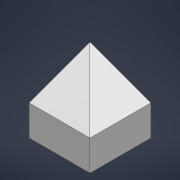
# Autodesk Inventor part: 110033226_ipt_35_中心城堡圍牆頂部_MIR
Saved by Autodesk Inventor 2022 (Build 260153000, 153)
## iProperties
Created: 2022-06-25
Part Number: 110033226_ipt_35_中心城堡圍牆頂部_MIR
Material: 一般
Document SubType Name: Modeling
Designer: User
Density: 1 g/cm^3
Appearance: 預設
Author: User
Autodesk Inventor part; units mm, degrees
ref_plane "YZ Plane" through (0, 0, 0) normal (1, 0, 0) x (0, 1, 0)
ref_plane "XZ Plane" through (0, 0, 0) normal (0, 1, 0) x (-1, 0, 0)
ref_plane "XY Plane" through (0, 0, 0) normal (0, 0, 1) x (1, 0, 0)
sketch "草圖1" plane through (0, 0, 0) normal (0, 1, 0) x (-1, 0, 0)
  line L0 (0, 0) -> (10, 0)
  line L1 (10, 0) -> (10, -10)
  line L2 (10, -10) -> (0, -10)
  line L3 (0, -10) -> (0, 0)
  circle A0 centre (7.5, -2.5) radius 1.7
  circle A1 centre (7.5, -7.5) radius 1.7
  circle A2 centre (2.5, -2.5) radius 1.7
  circle A3 centre (2.5, -7.5) radius 1.7
  dimension "d0" = 10
  dimension "d1" = 10
  dimension "d2" = 3.4
  dimension "d3" = 2.5
  dimension "d4" = 2.5
  dimension "d7" = 5
  dimension "d10" = 5
  constraints: 8 end point, 4 centre point, 2 horizontal, 2 parallel, 1 perpendicular, 1 vertical, 6 other
  measures "d0" distance of L1.end L2.end
  measures "d1" distance of L0.end L1.end
  measures "d2" diameter of A0
  measures "d3" distance from line of A0.centre L1
  measures "d4" distance from line of A0.centre L0
  measures "d7" distance of A0.centre A1.centre
  measures "d10" distance of A0.centre A2.centre
extrude "擠出1" add sketch "草圖1" against normal blind 5 contours L0 L1 L2 L3 | A0 | A1 | A2 | A3
sketch "草圖1 outline for 擠出2" plane through (0, 0, 0) normal (0, 1, 0) x (-1, 0, 0)
  line L0 (0, 0) -> (0, -10)
  line L1 (10, 0) -> (0, 0)
  line L2 (10, -10) -> (10, 0)
  line L3 (0, -10) -> (10, -10)
extrude "擠出2" add sketch "草圖1 outline for 擠出2" along normal blind 10 draft -30
sketch "草圖2" plane through (0, -5, 0) normal (0, -1, 0) x (1, 0, 0)
  circle A0 centre (-7.5, -7.5) radius 1.7 projected
  line L0 (-10, -10) -> (0, -10) projected
  line L1 (0, -10) -> (0, 0) projected
  line L2 (0, 0) -> (-10, 0) projected
  line L3 (-10, 0) -> (-10, -10) projected
extrude "擠出3" cut sketch "草圖2" against normal blind 1.5 contours A0
pattern_linear "矩形陣列1" count 2 spacing 5 along (0, 0, 1) count 2 spacing 5 along (1, 0, 0) of "擠出3"
